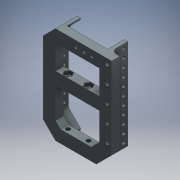
# Autodesk Inventor part: chassi_back_left
Saved by Autodesk Inventor 2016 (Build 200138000, 138)
## iProperties
Created: 2017-01-03
Part Number: chassi_back_left
Material: Generic
Document SubType Name: Modeling
Designer: hesaon
Density: 1 g/cm^3
Appearance: Default
Author: hesaon
Autodesk Inventor part; units mm, degrees
ref_plane "YZ Plane" through (0, 0, 0) normal (1, 0, 0) x (0, 1, 0)
ref_plane "XZ Plane" through (0, 0, 0) normal (0, 1, 0) x (-1, 0, 0)
ref_plane "XY Plane" through (0, 0, 0) normal (0, 0, 1) x (1, 0, 0)
sketch "Sketch1" plane through (0, 0, 0) normal (0, 1, 0) x (-1, 0, 0)
  line L0 (0, 117.0442) -> (0, 88.5)
  line L1 (0, 142.5) -> (-82.5, 142.5)
  line L2 (0, 0) -> (-60, 0)
  line L3 (-60, 0) -> (-82.5, 22.5)
  line L4 (-82.5, 142.5) -> (-82.5, 22.5)
  line L5 (-64.5, 124.5) -> (-7.4558, 124.5)
  line L6 (0, 88.5) -> (-64.5, 88.5)
  line L7 (-64.5, 29.9558) -> (-64.5, 70.5)
  line L8 (-64.5, 88.5) -> (-64.5, 124.5)
  line L9 (-52.5442, 18) -> (-64.5, 29.9558)
  line L10 (-45.5, 0) -> (0, 0)
  line L11 (-45.5, 0) -> (0, 0)
  line L12 (0, 0) -> (18, 18)
  line L13 (-7.4558, 18) -> (-52.5442, 18)
  line L14 (-64.5, 70.5) -> (0, 70.5)
  line L15 (0, 70.5) -> (0, 25.4558)
  line L16 (0, 25.4558) -> (-7.4558, 18)
  line L17 (0, 142.5) -> (18, 124.5)
  line L18 (18, 18) -> (18, 124.5)
  line L19 (0, 117.0442) -> (-7.4558, 124.5)
  point P0 (0, 0)
  dimension "d1" = 142.5
  dimension "d3" = 82.5
  dimension "d4" = 60
  dimension "d5" = 135
  dimension "d6" = 120
  dimension "d8" = 18
  dimension "d17" = 18
  dimension "d20" = 18
  dimension "d21" = 18
  dimension "d58" = 45.5
  dimension "d59" = 45.5
  dimension "d61" = 18
  dimension "d65" = 18
  dimension "d66" = 18
  dimension "d68" = 135
  dimension "d73" = 45
  dimension "d74" = 18
  dimension "d75" = 36
  dimension "d76" = 64.5
  dimension "d77" = 64.5
  dimension "d78" = 45
  dimension "d79" = 106.5
  constraints: 40 end point, 6 perpendicular, 4 horizontal, 4 vertical, 3 parallel, 1 coincident
  measures "d1" distance of L2.start L1.start
  measures "d3" distance of L1.start L1.end
  measures "d4" distance of L2.start L2.end
  measures "d5" angle of L2 L3
  measures "d6" distance of L3.end L1.end
  measures "d8" distance between parallel lines of L1 L5
  measures "d17" distance of L7.end L6.end
  measures "d20" distance between parallel lines of L4 L8
  measures "d21" distance between parallel lines of L3 L9
  measures "d58" distance of L2.start L10.start
  measures "d59" distance of L10.start L2.start
  measures "d61" distance between parallel lines of L2 L13
  measures "d65" distance between parallel lines of L16 L12
  measures "d66" distance between parallel lines of L4 L7
  measures "d68" angle of L13 L16
  measures "d73" angle of L0 L17
  measures "d74" distance between parallel lines of L17 L19
  measures "d75" distance between parallel lines of L5 L6
  measures "d76" distance between parallel lines of L8 L0
  measures "d77" distance between parallel lines of L7 L15
  measures "d78" angle of L12 L2
  measures "d79" distance of L17.end L12.end
extrude "Extrusion2" add sketch "Sketch1" along normal blind 12
sketch "Sketch7" plane through (0, 0, 0) normal (0, -1, 0) x (1, 0, 0)
  circle A0 centre (29.625, 133.5) radius 2.5
  circle A1 centre (41.25, 133.5) radius 2.5
  circle A2 centre (52.875, 133.5) radius 2.5
  line L0 (7.4558, 124.5) -> (64.5, 124.5) projected
  line L1 (0, 88.5) -> (0, 117.0442) projected
  line L2 (64.5, 124.5) -> (64.5, 88.5) projected
  point P0 (0, 0)
  dimension "d47" = 5
  dimension "d48" = 5
  dimension "d49" = 5
  dimension "d50" = 11.625
  dimension "d51" = 11.625
  dimension "d52" = 9
  dimension "d90" = 11.625
  constraints: 3 centre point, 2 horizontal alignment
  measures "d47" diameter of A0
  measures "d48" diameter of A1
  measures "d49" diameter of A2
  measures "d50" distance of A1.centre A0.centre
  measures "d51" distance of A1.centre A2.centre
  measures "d52" distance from line of L0 A0.centre
  measures "d90" distance from line of L2 A2.centre
extrude "Extrusion7" cut sketch "Sketch7" against normal up to next
sketch "Sketch8" plane through (60, 0, 0) normal (0, 0, -1) x (-1, 0, 0)
  line L0 (78, 0) -> (32.5, 0)
  line L1 (0, 0) -> (60, 0) projected
  circle A0 centre (47.5, 6) radius 3
  line L2 (32.5, 0) -> (32.5, 12)
  line L3 (0, 12) -> (60, 12) projected
  circle A1 centre (17.5, 6) radius 3
  dimension "d80" = 45.5
  dimension "d81" = 6
  dimension "d82" = 6
  dimension "d83" = 15
  dimension "d84" = 6
  dimension "d85" = 15
  dimension "d86" = 6
  constraints: 4 end point, 2 centre point, 2 point on line, 1 vertical
  measures "d80" distance of L0.start L0.end
  measures "d81" diameter of A0
  measures "d82" distance from line of L0 A0.centre
  measures "d83" distance from line of L2 A0.centre
  measures "d84" diameter of A1
  measures "d85" distance from line of A1.centre L2
  measures "d86" distance from line of L1 A1.centre
extrude "Extrusion8" cut sketch "Sketch8" against normal blind 88.5
sketch "Sketch9" plane through (0, 0, 0) normal (0, -1, 0) x (1, 0, 0)
  circle A0 centre (75.5, 35) radius 3
  line L0 (82.5, 142.5) -> (82.5, 22.5) projected
  circle A1 centre (75.5, 60) radius 3
  circle A2 centre (75.5, 85) radius 3
  circle A3 centre (75.5, 110) radius 3
  circle A4 centre (75.5, 135) radius 3
  point P0 (0, 0)
  dimension "d91" = 6
  dimension "d92" = 7
  dimension "d93" = 12.5
  dimension "d94" = 6
  dimension "d95" = 25
  dimension "d96" = 6
  dimension "d97" = 25
  dimension "d98" = 6
  dimension "d99" = 25
  dimension "d100" = 6
  dimension "d101" = 25
  constraints: 5 centre point, 4 vertical alignment
  measures "d91" diameter of A0
  measures "d92" distance from line of L0 A0.centre
  measures "d93" vertical distance of A0.centre L0.end
  measures "d94" diameter of A1
  measures "d95" distance of A1.centre A0.centre
  measures "d96" diameter of A2
  measures "d97" distance of A2.centre A1.centre
  measures "d98" diameter of A3
  measures "d99" distance of A2.centre A3.centre
  measures "d100" diameter of A4
  measures "d101" distance of A4.centre A3.centre
extrude "Extrusion9" cut sketch "Sketch9" against normal up to next
sketch "Sketch17" plane through (0, 0, 88.5) normal (0, 0, 1) x (1, 0, 0)
  circle A0 centre (12.5, 6) radius 3 projected
  line L0 (15.5022, 11.2) -> (18.5044, 6)
  line L1 (18.5044, 6) -> (15.5022, 0.8)
  line L2 (15.5022, 0.8) -> (9.4978, 0.8)
  line L3 (9.4978, 0.8) -> (6.4956, 6)
  line L4 (6.4956, 6) -> (9.4978, 11.2)
  line L5 (9.4978, 11.2) -> (15.5022, 11.2)
  circle A1 centre (42.5, 6) radius 3 projected
  line L6 (45.5022, 11.2) -> (48.5044, 6)
  line L7 (48.5044, 6) -> (45.5022, 0.8)
  line L8 (45.5022, 0.8) -> (39.4978, 0.8)
  line L9 (39.4978, 0.8) -> (36.4956, 6)
  line L10 (36.4956, 6) -> (39.4978, 11.2)
  line L11 (39.4978, 11.2) -> (45.5022, 11.2)
  line L12 (64.5, 12) -> (0, 12) projected
  point P0 (0, 0)
  point P1 (42.5, 11.2)
  dimension "d170" = 10.4
  dimension "d171" = 10.4
  constraints: 24 end point, 2 coincident, 1 midpoint, 1 parallel, 1 point on line, 26 other
  measures "d170" distance between parallel lines of L5 L2
  measures "d171" distance between parallel lines of L11 L8
extrude "Extrusion17" cut sketch "Sketch17" against normal blind 5
sketch "Sketch18" plane through (0, 12, 0) normal (0, 1, 0) x (1, 0, 0)
  circle A0 centre (75.5, -110) radius 3 projected
  circle A1 centre (75.5, -60) radius 3 projected
  circle A2 centre (75.5, -35) radius 3 projected
  circle A3 centre (75.5, -85) radius 3 projected
  circle A4 centre (75.5, -135) radius 3 projected
  circle A5 centre (41.25, -133.5) radius 2.5 projected
  circle A6 centre (29.625, -133.5) radius 2.5 projected
  circle A7 centre (52.875, -133.5) radius 2.5 projected
  line L0 (64.5, -70.5) -> (0, -70.5) projected
  line L1 (0, -70.5) -> (0, -25.4558) projected
  line L2 (0, -25.4558) -> (7.4558, -18) projected
  line L3 (7.4558, -18) -> (52.5442, -18) projected
  line L4 (52.5442, -18) -> (64.5, -29.9558) projected
  line L5 (64.5, -29.9558) -> (64.5, -70.5) projected
  line L6 (7.4558, -124.5) -> (0, -117.0442) projected
  line L7 (0, -117.0442) -> (0, -88.5) projected
  line L8 (0, -88.5) -> (64.5, -88.5) projected
  line L9 (64.5, -88.5) -> (64.5, -124.5) projected
  line L10 (64.5, -124.5) -> (7.4558, -124.5) projected
  line L11 (0, -142.5) -> (82.5, -142.5) projected
  line L12 (82.5, -142.5) -> (82.5, -22.5) projected
  line L13 (82.5, -22.5) -> (60, 0) projected
  line L14 (60, 0) -> (0, 0) projected
  line L15 (0, 0) -> (-18, -18) projected
  line L16 (-18, -18) -> (-18, -124.5) projected
  line L17 (-18, -124.5) -> (0, -142.5) projected
  line L18 (0, -142.5) -> (82.5, -142.5) projected
  line L19 (64.5, -142.5) -> (64.5, -4.5)
  line L20 (82.5, -22.5) -> (60, 0) projected
  line L21 (64.5, -70.5) -> (64.5, -29.9558) projected
  line L22 (64.5, -142.5) -> (69.5, -142.5)
  line L23 (69.5, -142.5) -> (69.5, -9.5)
  line L24 (64.5, -4.5) -> (69.5, -9.5)
  point P0 (0, 0)
  dimension "d174" = 5
  constraints: 8 end point, 5 point on line, 2 collinear, 1 perpendicular
  measures "d174" distance of L19.start L22.end
extrude "Extrusion18" add sketch "Sketch18" along normal blind 25 contours L5 L19 L13 L23 L11 L9
sketch "Sketch19" plane through (0, 12, 0) normal (0, 1, 0) x (1, 0, 0)
  circle A0 centre (75.5, -135) radius 3 projected
  line L0 (70.3, -131.9978) -> (75.5, -128.9956)
  line L1 (75.5, -128.9956) -> (80.7, -131.9978)
  line L2 (80.7, -131.9978) -> (80.7, -138.0022)
  line L3 (80.7, -138.0022) -> (75.5, -141.0044)
  line L4 (75.5, -141.0044) -> (70.3, -138.0022)
  line L5 (70.3, -138.0022) -> (70.3, -131.9978)
  circle A1 centre (75.5, -110) radius 3 projected
  line L6 (70.3, -106.9978) -> (75.5, -103.9956)
  line L7 (75.5, -103.9956) -> (80.7, -106.9978)
  line L8 (80.7, -106.9978) -> (80.7, -113.0022)
  line L9 (80.7, -113.0022) -> (75.5, -116.0044)
  line L10 (75.5, -116.0044) -> (70.3, -113.0022)
  line L11 (70.3, -113.0022) -> (70.3, -106.9978)
  circle A2 centre (75.5, -85) radius 3 projected
  line L12 (70.3, -81.9978) -> (75.5, -78.9956)
  line L13 (75.5, -78.9956) -> (80.7, -81.9978)
  line L14 (80.7, -81.9978) -> (80.7, -88.0022)
  line L15 (80.7, -88.0022) -> (75.5, -91.0044)
  line L16 (75.5, -91.0044) -> (70.3, -88.0022)
  line L17 (70.3, -88.0022) -> (70.3, -81.9978)
  line L18 (70.3, -63.0022) -> (70.3, -56.9978)
  line L19 (70.3, -56.9978) -> (75.5, -53.9956)
  line L20 (75.5, -53.9956) -> (80.7, -56.9978)
  line L21 (80.7, -56.9978) -> (80.7, -63.0022)
  line L22 (80.7, -63.0022) -> (75.5, -66.0044)
  line L23 (75.5, -66.0044) -> (70.3, -63.0022)
  line L24 (70.3, -38.0022) -> (70.3, -31.9978)
  line L25 (70.3, -31.9978) -> (75.5, -28.9956)
  line L26 (75.5, -28.9956) -> (80.7, -31.9978)
  line L27 (80.7, -31.9978) -> (80.7, -38.0022)
  line L28 (80.7, -38.0022) -> (75.5, -41.0044)
  line L29 (75.5, -41.0044) -> (70.3, -38.0022)
  circle A3 centre (75.5, -60) radius 3 projected
  circle A4 centre (75.5, -35) radius 3 projected
  line L30 (82.5, -142.5) -> (82.5, -22.5) projected
  point P0 (0, 0)
  point P1 (70.3, -110)
  point P2 (70.3, -85)
  dimension "d177" = 10.4
  dimension "d178" = 10.4
  dimension "d179" = 10.4
  dimension "d180" = 10.4
  dimension "d181" = 10.4
  constraints: 60 end point, 5 coincident, 3 parallel, 2 midpoint, 2 point on line, 65 other
  measures "d177" distance between parallel lines of L2 L5
  measures "d178" distance between parallel lines of L8 L11
  measures "d179" distance between parallel lines of L14 L17
  measures "d180" distance between parallel lines of L20 L23
  measures "d181" distance between parallel lines of L26 L29
extrude "Extrusion19" cut sketch "Sketch19" against normal blind 5
fillet "Fillet7" radius 8 1 edges at (69.5, 12, 76)
sketch "Sketch20" plane through (0, 12, 0) normal (0, 1, 0) x (1, 0, 0)
  line L0 (-18, -124.5) -> (0, -142.5) projected
  line L1 (0, -142.5) -> (5, -142.5)
  line L2 (0, -142.5) -> (82.5, -142.5) projected
  line L3 (0, -142.5) -> (-18, -124.5)
  line L4 (0, 0) -> (5, 0)
  line L5 (60, 0) -> (0, 0) projected
  line L6 (5, -140.4289) -> (-13, -122.4289)
  line L7 (-13, -122.4289) -> (-13, -20.0711)
  line L8 (-18, -18) -> (-18, -124.5) projected
  line L9 (-18, -124.5) -> (0, -142.5) projected
  line L10 (0, 0) -> (-18, -18) projected
  line L11 (5, -140.4289) -> (5, -142.5)
  line L12 (5, 0) -> (5, -2.0711)
  line L13 (-13, -20.0711) -> (5, -2.0711)
  line L14 (-18, -18) -> (0, 0)
  dimension "d185" = 5
  dimension "d186" = 5
  dimension "d187" = 5
  dimension "d190" = 5
  dimension "d192" = 5
  constraints: 18 end point, 3 parallel, 3 point on line, 1 perpendicular, 1 vertical
  measures "d185" distance of L0.end L1.end
  measures "d186" distance between parallel lines of L8 L7
  measures "d187" distance between parallel lines of L0 L6
  measures "d190" distance of L4.end L4.start
  measures "d192" distance between parallel lines of L10 L13
extrude "Extrusion20" add sketch "Sketch20" along normal blind 20
sketch "Sketch25" plane through (-18, 0, 18) normal (-1, 0, 0) x (0, 0, 1)
  line L0 (124.5, 0) -> (124.5, 32) projected
  line L1 (-18, 0) -> (-18, 32) projected
  line L2 (53.25, -34.9352) -> (53.25, 60.3708)
  circle A0 centre (47.25, 26) radius 2.5
  line L3 (0, 32) -> (106.5, 32) projected
  circle A1 centre (35.25, 26) radius 2.5
  circle A2 centre (23.25, 26) radius 2.5
  circle A3 centre (11.25, 26) radius 2.5
  circle A4 centre (59.25, 26) radius 2.5
  circle A5 centre (71.25, 26) radius 2.5
  circle A6 centre (83.25, 26) radius 2.5
  circle A7 centre (95.25, 26) radius 2.5
  dimension "d232" = 71.25
  dimension "d233" = 5
  dimension "d234" = 6
  dimension "d235" = 6
  dimension "d236" = 5
  dimension "d237" = 5
  dimension "d238" = 5
  dimension "d239" = 5
  dimension "d240" = 5
  dimension "d241" = 5
  dimension "d242" = 5
  dimension "d243" = 12
  dimension "d244" = 12
  dimension "d245" = 12
  dimension "d246" = 12
  dimension "d247" = 12
  dimension "d248" = 12
  dimension "d249" = 12
  constraints: 8 centre point, 7 horizontal alignment, 2 end point, 1 vertical
  measures "d232" distance between parallel lines of L2 L1
  measures "d233" diameter of A0
  measures "d234" distance from line of L2 A0.centre
  measures "d235" distance from line of L3 A0.centre
  measures "d236" diameter of A1
  measures "d237" diameter of A2
  measures "d238" diameter of A3
  measures "d239" diameter of A4
  measures "d240" diameter of A5
  measures "d241" diameter of A6
  measures "d242" diameter of A7
  measures "d243" distance of A0.centre A4.centre
  measures "d244" distance of A4.centre A5.centre
  measures "d245" distance of A6.centre A5.centre
  measures "d246" distance of A7.centre A6.centre
  measures "d247" distance of A1.centre A0.centre
  measures "d248" distance of A2.centre A1.centre
  measures "d249" distance of A3.centre A2.centre
extrude "Extrusion21" cut sketch "Sketch25" against normal blind 5
sketch "Sketch27" plane through (69.5, 37, 142.5) normal (1, 0, 0) x (0, 0, -1)
  circle A0 centre (6, -6) radius 2.5
  line L0 (0, -17) -> (0, 0) projected
  line L1 (0, 0) -> (133, 0) projected
  circle A1 centre (18, -6) radius 2.5
  circle A2 centre (30, -6) radius 2.5
  circle A3 centre (42, -6) radius 2.5
  circle A4 centre (54, -6) radius 2.5
  circle A5 centre (66, -6) radius 2.5
  circle A6 centre (78, -6) radius 2.5
  circle A7 centre (90, -6) radius 2.5
  circle A8 centre (102, -6) radius 2.5
  circle A9 centre (114, -6) radius 2.5
  circle A10 centre (126, -6) radius 2.5
  line L2 (133, -17) -> (133, 0) projected
  point P0 (142.5, -37)
  dimension "d252" = 5
  dimension "d253" = 6
  dimension "d254" = 6
  dimension "d255" = 5
  dimension "d256" = 5
  dimension "d257" = 5
  dimension "d258" = 5
  dimension "d259" = 5
  dimension "d260" = 12
  dimension "d261" = 12
  dimension "d262" = 12
  dimension "d263" = 12
  dimension "d264" = 12
  dimension "d265" = 5
  dimension "d266" = 5
  dimension "d267" = 5
  dimension "d268" = 5
  dimension "d269" = 12
  dimension "d270" = 12
  dimension "d271" = 12
  dimension "d272" = 12
  dimension "d273" = 12
  dimension "d274" = 6
  dimension "d280" = 5
  constraints: 11 centre point, 9 horizontal alignment
  measures "d252" diameter of A0
  measures "d253" distance from line of L0 A0.centre
  measures "d254" distance from line of A0.centre L1
  measures "d255" diameter of A1
  measures "d256" diameter of A2
  measures "d257" diameter of A3
  measures "d258" diameter of A4
  measures "d259" diameter of A5
  measures "d260" distance of A1.centre A0.centre
  measures "d261" distance of A2.centre A1.centre
  measures "d262" distance of A3.centre A2.centre
  measures "d263" distance of A4.centre A3.centre
  measures "d264" distance of A5.centre A4.centre
  measures "d265" diameter of A6
  measures "d266" diameter of A7
  measures "d267" diameter of A8
  measures "d268" diameter of A9
  measures "d269" distance of A6.centre A5.centre
  measures "d270" distance of A7.centre A6.centre
  measures "d271" distance of A8.centre A7.centre
  measures "d272" distance of A9.centre A8.centre
  measures "d273" distance of A10.centre A9.centre
  measures "d274" distance from line of L1 A7.centre
  measures "d280" diameter of A10
extrude "Extrusion22" cut sketch "Sketch27" against normal blind 5
fillet "Fillet8" radius 8 1 edges at (-13, 12, 71.25)
fillet "Fillet9" radius 8 1 edges at (0, 12, 7.0711)
fillet "Fillet10" radius 8 1 edges at (0, 12, 135.4289)
body "Solid2"
